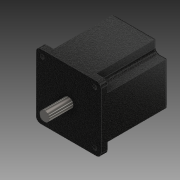
# Autodesk Inventor part: 1224_Stepper Motor_V1
Saved by Autodesk Inventor 2020 (Build 240168000, 168)
## iProperties
Created: 2019-09-12
Part Number: 1224_Stepper Motor_V1
Material: Generic
Document SubType Name: Modeling
Designer: MPI
Density: 1 g/cm^3
Appearance: Black Cast
Author: MPI
Autodesk Inventor part; units mm, degrees
ref_plane "YZ Plane" through (0, 0, 0) normal (1, 0, 0) x (0, 1, 0)
ref_plane "XZ Plane" through (0, 0, 0) normal (0, 1, 0) x (-1, 0, 0)
ref_plane "XY Plane" through (0, 0, 0) normal (0, 0, 1) x (1, 0, 0)
sketch "Sketch1" plane through (0, 0, 0) normal (0, 1, 0) x (-1, 0, 0)
  line L0 (36.926, 42.926) -> (-36.926, 42.926)
  line L1 (-42.926, 36.926) -> (-42.926, -36.926)
  line L2 (-36.926, -42.926) -> (36.926, -42.926)
  line L3 (42.926, -36.926) -> (42.926, 36.926)
  line L4 (55, 0) -> (-75, 0) construction
  line L5 (0, 74) -> (0, -88) construction
  arc A0 (42.926, 36.926) -> (36.926, 42.926) centre (36.926, 36.926) ccw
  arc A1 (36.926, -42.926) -> (42.926, -36.926) centre (36.926, -36.926) ccw
  arc A2 (-42.926, -36.926) -> (-36.926, -42.926) centre (-36.926, -36.926) ccw
  arc A3 (-36.926, 42.926) -> (-42.926, 36.926) centre (-36.926, 36.926) ccw
  circle A4 centre (34.798, 34.798) radius 2.7559
  circle A5 centre (34.798, -34.798) radius 2.7559
  circle A6 centre (-34.798, -34.798) radius 2.7559
  circle A7 centre (-34.798, 34.798) radius 2.7559
  point P0 (0, 0)
  point P1 (42.926, 42.926)
  point P2 (42.926, -42.926)
  point P3 (42.926, 0)
  point P4 (0, -42.926)
  dimension "d0" = 85.852
  dimension "d1" = 6
  dimension "d5" = 5.5118
  dimension "d6" = 69.596
  dimension "d7" = 69.596
  dimension "d8" = 69.596
  dimension "d9" = 69.596
  dimension "d10" = 34.798
  dimension "d11" = 34.798
  constraints: 12 end point, 8 centre point, 8 point on circle, 8 point on line, 8 tangent, 6 equal radius, 2 horizontal, 2 midpoint, 2 parallel, 2 perpendicular, 1 vertical
  measures "d0" distance of point (42.926, -42.926) point (42.926, 42.926)
  measures "d1" radius of A0
  measures "d5" diameter of A7
  measures "d6" distance of A5.centre A4.centre
  measures "d7" distance of A6.centre A5.centre
  measures "d8" distance of A7.centre A6.centre
  measures "d9" distance of A7.centre A4.centre
  measures "d10" horizontal distance of point (0, 0) A4.centre
  measures "d11" horizontal distance of point (0, 0) A4.centre
extrude "Extrusion1" add sketch "Sketch1" along normal blind 8.382
sketch "Sketch2" plane through (0, 8.382, 0) normal (0, 1, 0) x (1, 0, 0)
  line L0 (42.926, -28) -> (42.926, 28)
  line L1 (-42.926, 28) -> (-42.926, -28)
  line L2 (-28, -42.926) -> (28, -42.926)
  line L3 (28, 42.926) -> (-28, 42.926)
  line L4 (-42.926, 36.926) -> (-42.926, -36.926) projected
  line L5 (36.926, 42.926) -> (-36.926, 42.926) projected
  line L6 (42.926, -36.926) -> (42.926, 36.926) projected
  line L7 (-36.926, -42.926) -> (36.926, -42.926) projected
  line L8 (-42.926, -28) -> (-33, -28)
  line L9 (33, -28) -> (42.926, -28)
  line L10 (-28, 42.926) -> (-28, 33)
  line L11 (-28, -33) -> (-28, -42.926)
  line L12 (42.926, 28) -> (33, 28)
  line L13 (-33, 28) -> (-42.926, 28)
  line L14 (28, -42.926) -> (28, -33)
  line L15 (28, 33) -> (28, 42.926)
  arc A0 (33, -28) -> (28, -33) centre (33, -33) ccw
  arc A1 (-28, -33) -> (-33, -28) centre (-33, -33) ccw
  arc A2 (-33, 28) -> (-28, 33) centre (-33, 33) ccw
  arc A3 (28, 33) -> (33, 28) centre (33, 33) ccw
  point P0 (0, 0)
  dimension "d14" = 56
  dimension "d16" = 56
  dimension "d18" = 5
  dimension "d30" = 28
  dimension "d31" = 28
  constraints: 24 end point, 10 parallel, 8 collinear, 8 point on circle, 8 tangent, 4 centre point, 4 perpendicular, 3 equal radius, 3 horizontal
  measures "d14" distance of L3.start L3.end
  measures "d16" distance of L1.start L1.end
  measures "d18" radius of A0
  measures "d30" distance from line of point (0, 0) L8
  measures "d31" distance from line of point (0, 0) L15
extrude "Extrusion2" add sketch "Sketch2" along normal blind 80.01
fillet "Fillet1" radius 3 16 edges at (29.4645, 88.392, 29.4645) (28, 88.392, 37.963) (37.963, 88.392, 28) (42.926, 88.392, 0) (0, 88.392, -42.926) (-42.926, 88.392, 0) (-28, 88.392, 37.963) (-37.963, 88.392, 28) (-29.4645, 88.392, 29.4645) (0, 88.392, 42.926) (29.4645, 88.392, -29.4645) (28, 88.392, -37.963) (37.963, 88.392, -28) (-29.4645, 88.392, -29.4645) (-28, 88.392, -37.963) (-37.963, 88.392, -28)
sketch "Sketch3" plane through (0, 0, 0) normal (0, -1, 0) x (1, 0, 0)
  circle A0 centre (0, 0) radius 6.35
  dimension "d22" = 12.7
  constraints: 1 centre point, 1 coincident
  measures "d22" diameter of A0
extrude "Extrusion3" add sketch "Sketch3" along normal blind 31.75
body "Solid1"
